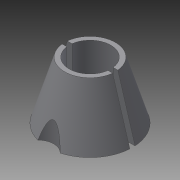
# Autodesk Inventor part: shaft collar
Saved by Autodesk Inventor 2014 (Build 180170000, 170)
## iProperties
Created: 2017-06-15
Part Number: shaft collar
Material: Generic
Document SubType Name: Modeling
Designer: RMcComber
Density: 1 g/cm^3
Appearance: Default
Author: RMcComber
Autodesk Inventor part; units mm, degrees
ref_plane "YZ Plane" through (0, 0, 0) normal (1, 0, 0) x (0, 1, 0)
ref_plane "XZ Plane" through (0, 0, 0) normal (0, 1, 0) x (-1, 0, 0)
ref_plane "XY Plane" through (0, 0, 0) normal (0, 0, 1) x (1, 0, 0)
sketch "Sketch1" plane through (0, 0, 0) normal (1, 0, 0) x (0, 1, 0)
  line L0 (0, 0) -> (4, 0) construction
  line L1 (4, 0) -> (4, 7)
  line L2 (4, 7) -> (4.9, 7)
  line L3 (4.9, 7) -> (7, 0)
  line L4 (7, 0) -> (4, 0)
  line L5 (4, 7) -> (4, 10) construction
  line L6 (4, 10) -> (4.9, 7) construction
  line L7 (4, 0) -> (4, -4)
  line L8 (4, -4) -> (8.2, -4)
  line L9 (8.2, -4) -> (7, 0)
  line L10 (0, 0) -> (0, 5.7266)
  dimension "d0" = 3
  dimension "d1" = 4
  dimension "d2" = 10
  dimension "d3" = 7
  dimension "d4" = 4
  constraints: 22 end point, 5 perpendicular, 3 collinear, 1 horizontal, 1 parallel
  measures "d0" distance of L3.end L0.end
  measures "d1" distance of L0.start L0.end
  measures "d2" distance from line of L5.end L4
  measures "d3" distance of L0.end L1.end
  measures "d4" distance of L0.end L7.end
revolve "Revolution1" add sketch "Sketch1" angle 360 about axis through (0, 0, 0) along (0, 0, 1)
sketch "Sketch2" plane through (0, 0, 7) normal (0, 0, 1) x (1, 0, 0)
  circle A0 centre (0, 0) radius 4.9 projected
  line L0 (10, -0.5) -> (-10, -0.5)
  line L1 (-10, -0.5) -> (-10, 0.5)
  line L2 (-10, 0.5) -> (10, 0.5)
  line L3 (10, 0.5) -> (10, -0.5)
  line L4 (10, -0.5) -> (-10, 0.5) construction
  line L5 (-10, -0.5) -> (10, 0.5) construction
  dimension "d6" = 1
  dimension "d7" = 20
  constraints: 12 end point, 2 midpoint, 2 parallel, 1 horizontal, 1 perpendicular
  measures "d6" distance of L0.end L1.end
  measures "d7" distance of L1.end L2.end
extrude "Extrusion1" cut sketch "Sketch2" against normal through all contours A0 L0 L2 | A0 L2 L3 L0 | A0 L0 L1 L2
sketch "Sketch3" plane through (0, 0, -4) normal (0, 0, -1) x (-1, 0, 0)
  arc A0 (-3.9686, -0.5) -> (3.9686, -0.5) centre (0, 0) ccw projected
  line L0 (-3.9686, -0.5) -> (-8.1847, -0.5) projected
  line L1 (0, 10) -> (0, -10)
  circle A1 centre (0, 10) radius 3
  circle A2 centre (0, -10) radius 3
  dimension "d10" = 20
  dimension "d11" = 6
  constraints: 3 coincident, 2 centre point, 2 end point, 1 equal radius, 1 midpoint, 1 perpendicular
  measures "d10" distance of L1.start L1.end
  measures "d11" diameter of A1
extrude "Extrusion2" cut sketch "Sketch3" against normal through all
body "Solid1"
